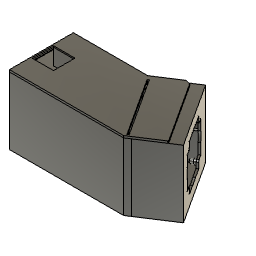
Spectroscope v11 (Autodesk Fusion 360 design; units mm, degrees)
Autodesk Fusion 360 part; units mm, degrees
(part 1 of 2)
sketch "Spectroscope Base" plane through (0, 0, 0) normal (0, 0, 1) x (1, 0, 0) in component "Spectrometer"
  line L0 (0, 0) -> (72, 0)
  line L1 (72, 0) -> (85.888295, -21.386099)
  line L2 (72, 0) -> (97.5, 0) construction
  line L3 (72, 0) -> (58.111705, 21.386099)
  line L4 (58.111705, 21.386099) -> (58.614907, 21.712883)
  line L5 (58.111705, 21.386099) -> (57.608502, 21.059316)
  line L6 (57.608502, 21.059316) -> (85.385093, -21.712883)
  line L7 (85.385093, -21.712883) -> (86.391498, -21.059316)
  line L8 (86.391498, -21.059316) -> (58.614907, 21.712883)
  line L9 (0, 0) -> (0, 23.787847)
  line L10 (0, 0) -> (0, -23.787847)
  line L11 (72, 0) -> (73.761208, 1.143742)
  line L12 (73.761208, 1.143742) -> (59.055954, 23.787847)
  line L13 (59.055954, 23.787847) -> (55.533538, 21.500363)
  line L14 (55.533538, 21.500363) -> (84.944046, -23.787847)
  line L15 (84.944046, -23.787847) -> (88.466462, -21.500363)
  line L16 (88.466462, -21.500363) -> (73.761208, 1.143742)
  line L17 (0, 23.787847) -> (59.055954, 23.787847)
  line L18 (0, -23.787847) -> (84.944046, -23.787847)
  line L19 (0, 0) -> (1.5, 0)
  line L20 (1.5, 0) -> (1.5, 22.287847)
  line L21 (1.5, 22.287847) -> (56.746157, 22.287847)
  line L22 (1.5, 0) -> (1.5, -22.287847)
  line L23 (1.5, -22.287847) -> (83.969934, -22.287847)
  line L24 (1.5, 0) -> (16.5, 0)
  line L25 (16.5, 0) -> (16.5, 7.5)
  line L26 (16.5, 7.5) -> (1.5, 7.5)
  line L27 (16.5, 0) -> (16.5, -7.5)
  line L28 (16.5, -7.5) -> (1.5, -7.5)
  line L29 (16.5, 0) -> (17.75, 0)
  line L30 (17.75, 0) -> (17.75, 8.75)
  line L31 (17.75, 8.75) -> (1.5, 8.75)
  line L32 (17.75, 0) -> (17.75, -8.75)
  line L33 (17.75, -8.75) -> (1.5, -8.75)
  line L34 (1.5, 0) -> (1.5, 1.469227)
  line L35 (1.5, 0) -> (1.5, 0.5)
  line L36 (1.5, 0.5) -> (0, 0.5)
  line L37 (1.5, 0) -> (1.5, -0.5)
  line L38 (1.5, -0.5) -> (0, -0.5)
  line L39 (0, -0.5) -> (0, 0.5)
  line L40 (58.111705, 21.386099) -> (60.8349, 17.192747)
  line L41 (60.8349, 17.192747) -> (62.596108, 18.336489)
  line L42 (60.8349, 17.192747) -> (59.073692, 16.049005)
  line L43 (85.888295, -21.386099) -> (83.1651, -17.192747)
  line L44 (83.1651, -17.192747) -> (81.403892, -18.336489)
  line L45 (83.1651, -17.192747) -> (84.926308, -16.049005)
  line L46 (55.533538, 21.500363) -> (55.02214, 22.287847)
  dimension "d1" = 72
  dimension "d3" = 25.5
  dimension "d4" = 25.5
  dimension "d9" = 123
  dimension "d10" = 0.6
  dimension "d11" = 0.6
  dimension "d12" = 51
  dimension "d13" = 1.2
  dimension "d14" = 51
  dimension "d18" = 23.787847
  dimension "d19" = 23.787847
  dimension "d22" = 2.1
  dimension "d23" = 27
  dimension "d24" = 4.2
  dimension "d25" = 90
  dimension "d26" = 54
  dimension "d27" = 4.2
  dimension "d28" = 27
  dimension "d29" = 1.5
  dimension "d30" = 22.287847
  dimension "d31" = 90
  dimension "d32" = 22.287847
  dimension "d34" = 15
  dimension "d35" = 7.5
  dimension "d36" = 15
  dimension "d37" = 7.5
  dimension "d38" = 15
  dimension "d40" = 1.25
  dimension "d41" = 8.75
  dimension "d42" = 16.25
  dimension "d43" = 8.75
  dimension "d44" = 16.25
  dimension "d46" = 0.5
  dimension "d47" = 1.5
  dimension "d48" = 0.5
  dimension "d49" = 1.5
  dimension "d50" = 1
  dimension "d52" = 5
  dimension "d53" = 2.1
  dimension "d54" = 2.1
  dimension "d55" = 5
  dimension "d56" = 2.1
  dimension "d57" = 2.1
  constraint coincident L0.start L9.start
  constraint horizontal L0
  constraint horizontal L2
  constraint parallel L1 L3
  constraint perpendicular L3 L4
  constraint perpendicular L3 L5
  constraint perpendicular L5 L6
  constraint perpendicular L1 L7
  constraint perpendicular L4 L8
  constraint perpendicular L0 L9
  constraint perpendicular L0 L10
  constraint perpendicular L6 L11
  constraint perpendicular L11 L12
  constraint perpendicular L13 L14
  constraint perpendicular L14 L15
  constraint perpendicular L11 L16
  constraint perpendicular L9 L19
  constraint perpendicular L17 L20
  constraint perpendicular L0 L22
  constraint horizontal L23
  constraint horizontal L24
  constraint vertical L25
  constraint horizontal L26
  constraint perpendicular L24 L27
  constraint perpendicular L27 L28
  constraint perpendicular L25 L29
  constraint perpendicular L29 L30
  constraint perpendicular L20 L31
  constraint perpendicular L29 L32
  constraint perpendicular L22 L33
  constraint perpendicular L19 L35
  constraint perpendicular L9 L36
  constraint perpendicular L36 L37
  constraint perpendicular L10 L38
  constraint perpendicular L36 L39
  constraint perpendicular L5 L40
  constraint perpendicular L12 L41
  constraint perpendicular L6 L42
  constraint perpendicular L7 L43
  constraint perpendicular L6 L44
  constraint perpendicular L43 L45
  constraint perpendicular L13 L46
  measures "d1" distance of L0.start L0.end
  measures "d9" angle of L0 L1
  measures "d25" angle of L12 L13
  measures "d29" distance of L0.start L19.end
  measures "d31" angle of L20 L21
  measures "d34" distance of L19.end L24.end
  measures "d35" distance of L24.end L25.end
  measures "d36" distance of L25.end L26.end
  measures "d37" distance of L24.end L27.end
  measures "d38" distance of L27.end L28.end
  measures "d40" distance of L24.end L29.end
  measures "d41" distance of L29.end L30.end
  measures "d42" distance of L30.end L31.end
  measures "d43" distance of L29.end L32.end
  measures "d44" distance of L32.end L33.end
  measures "d46" distance of L19.end L35.end
  measures "d47" distance of L35.end L36.end
  measures "d48" distance of L19.end L37.end
  measures "d49" distance of L37.end L38.end
  measures "d50" distance of L38.end L36.end
sketch "Sketch2" plane through (0, 0, 0) normal (1, 0, 0) x (0, 1, 0) in component "Spectrometer"
  line L0 (0, 0) -> (0, 50)
  line L1 (0, 50) -> (23.787847, 50)
  line L2 (0, 50) -> (-23.787847, 50)
  line L3 (-23.787847, 50) -> (-23.787847, 0)
  line L4 (23.787847, 50) -> (23.787847, 0)
  line L5 (23.787847, 0) -> (-23.787847, 0)
  line L6 (0, 0) -> (0, 1.5)
  dimension "d62" = 50
  dimension "d63" = 23.787847
  dimension "d64" = 23.787847
  dimension "d65" = 50
  dimension "d66" = 50
  dimension "d67" = 47.575695
  dimension "d68" = 1.5
  constraint coincident L0.start L6.start
  constraint vertical L0
  constraint perpendicular L0 L1
  constraint perpendicular L0 L2
  constraint perpendicular L2 L3
  constraint perpendicular L1 L4
  constraint perpendicular L4 L5
  constraint perpendicular L5 L6
  measures "d62" distance of L0.start L0.end
  measures "d68" distance of L0.start L6.end
ref_plane "WorkPlane1" through (71.496798, -0.326783, 0) normal (-0.838671, -0.544639, 0) x (0.544639, -0.838671, 0) in component "Spectrometer"
sketch "Camera Mount" plane through (71.496798, -0.326783, 0) normal (-0.838671, -0.544639, 0) x (0.544639, -0.838671, 0) in component "Spectrometer"
  line L0 (0, 0) -> (-27, 0)
  line L1 (0, 0) -> (0, 25)
  line L2 (0, 25) -> (14.000714, 39.000714)
  line L3 (0, 25) -> (19.8, 25) construction
  circle A0 centre (14.000714, 39.000714) radius 1.25
  line L4 (14.000714, 39.000714) -> (16.998847, 41.998847)
  circle A1 centre (16.998847, 41.998847) radius 1.25
  circle A2 centre (-16.998847, 41.998847) radius 1.25
  line L5 (-14.000714, 39.000714) -> (-16.998847, 41.998847)
  circle A3 centre (-14.000714, 39.000714) radius 1.25
  line L6 (0, 25) -> (-14.000714, 39.000714)
  circle A4 centre (-16.998847, 8.001153) radius 1.25
  line L7 (-14.000714, 10.999286) -> (-16.998847, 8.001153)
  circle A5 centre (-14.000714, 10.999286) radius 1.25
  line L8 (0, 25) -> (-14.000714, 10.999286)
  circle A6 centre (16.998847, 8.001153) radius 1.25
  line L9 (14.000714, 10.999286) -> (16.998847, 8.001153)
  circle A7 centre (14.000714, 10.999286) radius 1.25
  line L10 (0, 25) -> (14.000714, 10.999286)
  line L11 (-19.5, 5.5) -> (19.5, 5.5)
  line L12 (19.5, 5.5) -> (19.5, 44.5)
  line L13 (19.5, 44.5) -> (-19.5, 44.5)
  line L14 (-19.5, 44.5) -> (-19.5, 5.5)
  line L15 (-19.5, 5.5) -> (19.5, 44.5) construction
  line L16 (19.5, 5.5) -> (-19.5, 44.5) construction
  line L17 (27, 50) -> (-27, 50)
  line L18 (-27, 50) -> (-27, 0)
  line L19 (-27, 0) -> (27, 0)
  line L20 (27, 0) -> (27, 50)
  line L21 (27, 50) -> (-27, 0) construction
  line L22 (-27, 50) -> (27, 0) construction
  circle A8 centre (16.998847, 41.998847) radius 1.75
  circle A9 centre (14.000714, 39.000714) radius 1.75
  circle A10 centre (-16.998847, 41.998847) radius 1.75
  circle A11 centre (-14.000714, 39.000714) radius 1.75
  circle A12 centre (-16.998847, 8.001153) radius 1.75
  circle A13 centre (-14.000714, 10.999286) radius 1.75
  circle A14 centre (16.998847, 8.001153) radius 1.75
  circle A15 centre (14.000714, 10.999286) radius 1.75
  line L23 (-14.000714, 10.999286) -> (-6.750714, 10.999286)
  line L24 (-11.750714, 7.999286) -> (-1.750714, 7.999286)
  line L25 (-1.750714, 7.999286) -> (-1.750714, 13.999286)
  line L26 (-1.750714, 13.999286) -> (-11.750714, 13.999286)
  line L27 (-11.750714, 13.999286) -> (-11.750714, 7.999286)
  line L28 (-11.750714, 7.999286) -> (-1.750714, 13.999286) construction
  line L29 (-1.750714, 7.999286) -> (-11.750714, 13.999286) construction
  line L30 (-17.000714, 13.249286) -> (-11.000714, 23.249286) construction
  line L31 (-11.000714, 13.249286) -> (-17.000714, 13.249286)
  line L32 (-11.000714, 23.249286) -> (-11.000714, 13.249286)
  line L33 (-17.000714, 23.249286) -> (-11.000714, 13.249286) construction
  line L34 (-17.000714, 13.249286) -> (-17.000714, 23.249286)
  line L35 (-17.000714, 23.249286) -> (-11.000714, 23.249286)
  line L36 (-14.000714, 10.999286) -> (-14.000714, 18.249286)
  line L37 (-11.750714, 13.999286) -> (-11.000714, 14.749286)
  line L38 (-11.750714, 13.999286) -> (-10.690054, 13.999286) construction
  line L39 (-11.750714, 13.999286) -> (-12.500714, 13.249286)
  line L40 (-11.000714, 13.249286) -> (-10.250714, 13.999286)
  line L41 (-11.000714, 13.249286) -> (-11.750714, 12.499286)
  line L42 (11.750714, 7.999286) -> (1.750714, 13.999286) construction
  line L43 (11.000714, 23.249286) -> (11.000714, 13.249286)
  line L44 (17.000714, 23.249286) -> (11.000714, 13.249286) construction
  line L45 (11.000714, 13.249286) -> (11.000714, 14.309946) construction
  line L46 (11.750714, 7.999286) -> (1.750714, 7.999286)
  line L47 (11.000714, 13.249286) -> (17.000714, 13.249286)
  line L48 (-25, 52) -> (25, -2) construction
  line L49 (11.000714, 13.249286) -> (10.250714, 13.999286)
  line L50 (14.000714, 10.999286) -> (6.750714, 10.999286)
  line L51 (0, 25) -> (14.000714, 10.999286)
  line L52 (19.5, 5.5) -> (-19.5, 44.5) construction
  line L53 (1.750714, 7.999286) -> (1.750714, 13.999286)
  line L54 (1.750714, 13.999286) -> (11.750714, 13.999286)
  line L55 (11.000714, 13.249286) -> (11.750714, 12.499286)
  line L56 (11.750714, 13.999286) -> (11.750714, 7.999286)
  line L57 (1.750714, 7.999286) -> (11.750714, 13.999286) construction
  line L58 (11.750714, 13.999286) -> (11.000714, 14.749286)
  line L59 (17.000714, 13.249286) -> (17.000714, 23.249286)
  line L60 (14.000714, 10.999286) -> (14.000714, 18.249286)
  line L61 (17.000714, 13.249286) -> (11.000714, 23.249286) construction
  line L62 (17.000714, 23.249286) -> (11.000714, 23.249286)
  line L63 (11.750714, 13.999286) -> (12.500714, 13.249286)
  line L64 (17.000714, 36.750714) -> (11.000714, 26.750714) construction
  line L65 (1.750714, 36.000714) -> (11.750714, 36.000714)
  line L66 (1.750714, 42.000714) -> (11.750714, 36.000714) construction
  line L67 (11.750714, 36.000714) -> (10.690054, 36.000714) construction
  line L68 (17.000714, 36.750714) -> (17.000714, 26.750714)
  line L69 (11.750714, 36.000714) -> (11.750714, 42.000714)
  line L70 (-27, 0) -> (27, 50) construction
  line L71 (11.750714, 36.000714) -> (11.000714, 35.250714)
  line L72 (14.000714, 39.000714) -> (14.000714, 31.750714)
  line L73 (0, 25) -> (14.000714, 39.000714)
  line L74 (19.5, 44.5) -> (-19.5, 5.5) construction
  line L75 (17.000714, 26.750714) -> (11.000714, 26.750714)
  line L76 (11.000714, 26.750714) -> (11.000714, 36.750714)
  line L77 (11.750714, 36.000714) -> (12.500714, 36.750714)
  line L78 (11.000714, 36.750714) -> (17.000714, 36.750714)
  line L79 (17.000714, 26.750714) -> (11.000714, 36.750714) construction
  line L80 (11.000714, 36.750714) -> (10.250714, 36.000714)
  line L81 (11.750714, 42.000714) -> (1.750714, 42.000714)
  line L82 (14.000714, 39.000714) -> (6.750714, 39.000714)
  line L83 (11.750714, 42.000714) -> (1.750714, 36.000714) construction
  line L84 (1.750714, 42.000714) -> (1.750714, 36.000714)
  line L85 (11.000714, 36.750714) -> (11.750714, 37.500714)
  line L86 (-11.750714, 42.000714) -> (-1.750714, 36.000714) construction
  line L87 (-11.000714, 26.750714) -> (-11.000714, 36.750714)
  line L88 (-17.000714, 26.750714) -> (-11.000714, 36.750714) construction
  line L89 (-11.000714, 36.750714) -> (-11.000714, 35.690054) construction
  line L90 (-11.750714, 42.000714) -> (-1.750714, 42.000714)
  line L91 (-11.000714, 36.750714) -> (-17.000714, 36.750714)
  line L92 (25, -2) -> (-25, 52) construction
  line L93 (-11.000714, 36.750714) -> (-10.250714, 36.000714)
  line L94 (-14.000714, 39.000714) -> (-6.750714, 39.000714)
  line L95 (0, 25) -> (-14.000714, 39.000714)
  line L96 (-19.5, 44.5) -> (19.5, 5.5) construction
  line L97 (-1.750714, 42.000714) -> (-1.750714, 36.000714)
  line L98 (-1.750714, 36.000714) -> (-11.750714, 36.000714)
  line L99 (-11.000714, 36.750714) -> (-11.750714, 37.500714)
  line L100 (-11.750714, 36.000714) -> (-11.750714, 42.000714)
  line L101 (-1.750714, 42.000714) -> (-11.750714, 36.000714) construction
  line L102 (-11.750714, 36.000714) -> (-11.000714, 35.250714)
  line L103 (-17.000714, 36.750714) -> (-17.000714, 26.750714)
  line L104 (-14.000714, 39.000714) -> (-14.000714, 31.750714)
  line L105 (-17.000714, 36.750714) -> (-11.000714, 26.750714) construction
  line L106 (-17.000714, 26.750714) -> (-11.000714, 26.750714)
  line L107 (-11.750714, 36.000714) -> (-12.500714, 36.750714)
  point P0 (0, 25)
  point P1 (0, 25)
  point P2 (-6.750714, 10.999286)
  point P3 (-14.000714, 18.249286)
  point P4 (6.750714, 10.999286)
  point P5 (14.000714, 18.249286)
  point P6 (14.000714, 31.750714)
  point P7 (6.750714, 39.000714)
  point P8 (-6.750714, 39.000714)
  point P9 (-14.000714, 31.750714)
  dimension "d70" = 27
  dimension "d71" = 25
  dimension "d73" = 45
  dimension "d74" = 19.8
  dimension "d80" = 2.5
  dimension "d82" = 4.24
  dimension "d83" = 2.5
  dimension "d85" = 360
  dimension "d87" = 39
  dimension "d88" = 39
  dimension "d89" = 54
  dimension "d90" = 50
  dimension "d92" = 3.5
  dimension "d93" = 3.5
  dimension "d95" = 360
  dimension "d96" = 7.25
  dimension "d97" = 10
  dimension "d98" = 6
  dimension "d99" = 45
  dimension "d101" = 360
  constraint coincident L0.start L1.start
  constraint horizontal L0
  constraint perpendicular L0 L1
  constraint horizontal L3
  constraint parallel L2 L4
  constraint horizontal L11
  constraint perpendicular L11 L12
  constraint parallel L11 L13
  constraint parallel L12 L14
  constraint coincident L15 P1
  constraint coincident L16 P1
  constraint coincident P1 P0
  constraint horizontal L17
  constraint perpendicular L17 L18
  constraint parallel L17 L19
  constraint parallel L18 L20
  constraint coincident L21 P1
  constraint coincident L22 P1
  constraint horizontal L23
  constraint horizontal L24
  constraint perpendicular L24 L25
  constraint parallel L24 L26
  constraint parallel L25 L27
  constraint horizontal L38
  constraint parallel L37 L39
  constraint parallel L39 L40
  constraint parallel L40 L41
  measures "d70" distance of L0.start L0.end
  measures "d71" distance of L0.start P0
  measures "d73" angle of L2 L3
  measures "d80" diameter of A0
  measures "d83" diameter of A1
  measures "d87" distance of L12.end L13.end
  measures "d88" distance of L11.end L12.end
  measures "d89" distance of L0.end L19.end
  measures "d90" distance of L17.end L0.end
  measures "d92" diameter of A8
  measures "d93" diameter of A9
  measures "d99" angle of L37 L38
extrude "Extrude1" add sketch "Spectroscope Base" along normal blind 1.5 contours L0 L9 L19 L20 L34 L35 L36 L39 | L0 L10 L19 L22 L37 L38 L39 | L0 L20 L24 L25 L26 L34 L35 | L0 L22 L24 L27 L28 L37 | L9 L13 L17 L20 L21 L34 L36 | L10 L14 L18 L22 L23 L38 | L0 L20 L25 L26 L29 L30 L31 | L0 L22 L27 L28 L29 L32 L33 | L0 L14 L20 L21 L30 L31 L46 | L0 L14 L22 L23 L32 L33 | L4 L5 L6 L8 L12 L13 L14 L41 L42 | L6 L7 L8 L14 L15 L16 L44 L45 | L0 L6 L14 L42 | L0 L6 L14 L44 | L8 L11 L12 L41 | L13 L21 L46 | L0 L3 L6 L42 | L0 L1 L6 L44 | L8 L11 L16 L45 | L3 L4 L8 L40 L41 | L3 L8 L11 L41 | L1 L8 L11 L45 | L3 L5 L6 L40 L42 | L1 L6 L7 L43 L44 | L1 L7 L8 L43 L45 picked at (0.5, 0.333333) picked at (0.5, -0.333333) picked at (11.5, 2.989742) picked at (11.5, -2.666667) picked at (0.5, 11.012616) picked at (28.814682, -23.287847) picked at (11.916667, 8.333333) picked at (11.916667, -8.333333) picked at (48.773243, 5.349668) picked at (56.216643, -9.02883) picked at (60.08899, 21.279073) picked at (86.594756, -19.536228) picked at (67.037439, 5.621988) picked at (74.061504, -6.112163) picked at (69.200838, 6.330018) picked at (55.767278, 22.025353) picked at (68.039827, 5.730916) picked at (75.315493, -5.839843) picked at (80.785273, -10.590409) picked at (60.094902, 18.699459) picked at (64.892068, 11.679687) picked at (75.889434, -5.621988) picked at (58.851702, 19.879387) picked at (83.905098, -18.699459) picked at (85.316032, -19.77046) makes body 1 in component "Spectrometer"
extrude "Extrude2" add sketch "Spectroscope Base" along normal blind 50 separate body contours L0 L9 L19 L20 L34 L35 L36 L39 | L0 L10 L19 L22 L37 L38 L39 | L9 L13 L17 L20 L21 L34 L36 | L10 L14 L18 L22 L23 L38 | L4 L5 L6 L8 L12 L13 L14 L41 L42 | L6 L7 L8 L14 L15 L16 L44 L45 | L13 L21 L46 picked at (0.5, 0.333333) picked at (0.5, -0.333333) picked at (0.5, 11.012616) picked at (28.814682, -23.287847) picked at (60.08899, 21.279073) picked at (86.594756, -19.536228) picked at (55.767278, 22.025353) makes body 2 in component "Spectrometer"
extrude "Extrude3" add sketch "Spectroscope Base" along normal blind 7.5 contours L0 L20 L25 L26 L29 L30 L31 | L0 L22 L27 L28 L29 L32 L33 | L0 L6 L14 L42 | L0 L6 L14 L44 | L8 L11 L12 L41 | L8 L11 L16 L45 picked at (11.916667, 8.333333) picked at (11.916667, -8.333333) picked at (67.037439, 5.621988) picked at (74.061504, -6.112163) picked at (69.200838, 6.330018) picked at (80.785273, -10.590409) bodies 1 2 in component "Spectrometer"
extrude "Extrude4" cut sketch "Spectroscope Base" along normal blind 12 from surface at 19 contours L0 L9 L19 L20 L34 L35 L36 L39 | L0 L10 L19 L22 L37 L38 L39 picked at (0.5, 0.333333) picked at (0.5, -0.333333) bodies 1 in component "Spectrometer"
extrude "Extrude5" add sketch "Camera Mount" along normal blind 1.5 separate body contours L0 L17 L18 L19 L20 | L2 L73 L76 L78 | L2 L65 L69 L73 | L65 L71 L76 | L65 L76 L80 | L2 A9 L69 L73 L82 | L69 L77 L78 | L69 L78 L85 | L2 A9 L72 L73 L78 | L2 A0 A9 L73 L82 | L2 A0 A9 L72 L73 | L2 A0 L73 L82 | L2 A0 L72 L73 | A0 L4 A9 L82 | A0 L4 A9 L72 | A0 L4 L82 | A0 L4 L72 | A1 | A2 | L5 A3 L104 | A3 L6 L94 L95 | L5 A3 L94 | A3 L6 L95 L104 | L5 A3 A11 L104 | L5 A3 A11 L94 | A3 L6 A11 L95 L104 | A3 L6 A11 L94 L95 | L6 A11 L94 L95 L100 | L6 A11 L91 L95 L104 | L6 L87 L91 L95 | L91 L99 L100 | L91 L100 L107 | L6 L95 L98 L100 | L87 L93 L98 | L87 L98 L102 | A4 | L7 A5 L23 | A5 L8 L36 | A5 L8 L23 | L7 A5 L36 | L7 A5 A13 L23 | L7 A5 A13 L36 | A5 L8 A13 L23 | A5 L8 A13 L36 | L8 A13 L31 L36 | L8 A13 L23 L27 | L8 L26 L27 | L27 L31 L39 | L27 L31 L41 | L8 L31 L32 | L26 L32 L37 | L26 L32 L40 | A6 | L9 A7 L60 | A7 L10 L50 L51 | L9 A7 L50 | A7 L10 L51 L60 | L9 A7 A15 L60 | L9 A7 A15 L50 | A7 L10 A15 L51 L60 | A7 L10 A15 L50 L51 | L10 A15 L50 L51 L56 | L10 A15 L47 L51 L60 | L10 L43 L47 L51 | L47 L55 L56 | L47 L56 L63 | L10 L51 L54 L56 | L43 L49 L54 | L43 L54 L58 | L11 L12 L13 L14 | A8 | A10 | A12 | A14 picked at (-24.5, 31.5) picked at (11.250714, 36.500714) picked at (11.500714, 36.250714) picked at (11.250714, 35.750714) picked at (10.750714, 36.250714) picked at (11.937258, 38.349736) picked at (12.000714, 36.500714) picked at (11.500714, 37.000714) picked at (13.349736, 36.937258) picked at (12.422371, 38.924574) picked at (13.924574, 37.422371) picked at (13.170946, 38.946328) picked at (13.946328, 38.170946) picked at (14.163585, 40.571634) picked at (15.47005, 38.420955) picked at (13.225327, 39.299814) picked at (14.812929, 38.824028) picked at (17.295564, 42.324189) picked at (-17.550973, 42.311234) picked at (-14.82554, 39.102447) picked at (-13.254921, 38.63293) picked at (-13.345539, 39.512018) picked at (-13.63293, 38.254921) picked at (-15.456712, 39.612586) picked at (-12.516447, 39.540406) picked at (-13.100286, 37.702179) picked at (-12.513378, 38.467053) picked at (-11.937258, 38.349736) picked at (-13.349736, 36.937258) picked at (-11.250714, 36.500714) picked at (-11.500714, 37.000714) picked at (-12.000714, 36.500714) picked at (-11.500714, 36.250714) picked at (-10.750714, 36.250714) picked at (-11.250714, 35.750714) picked at (-16.820738, 8.324208) picked at (-13.225327, 10.700186) picked at (-13.946328, 11.829054) picked at (-13.185143, 11.161513) picked at (-14.82554, 10.897553) picked at (-12.428204, 10.852555) picked at (-15.530734, 10.607676) picked at (-12.445813, 11.28079) picked at (-12.979474, 12.205118) picked at (-13.349736, 13.062742) picked at (-11.937258, 11.650264) picked at (-11.500714, 13.749286) picked at (-12.000714, 13.499286) picked at (-11.500714, 12.999286) picked at (-11.250714, 13.499286) picked at (-11.250714, 14.249286) picked at (-10.750714, 13.749286) picked at (17.345998, 8.256868) picked at (14.666132, 11.497411) picked at (13.213295, 11.266578) picked at (13.171891, 10.938148) picked at (13.63293, 11.745079) picked at (15.47005, 11.579045) picked at (12.428204, 10.852555) picked at (13.870188, 12.574064) picked at (12.445813, 11.28079) picked at (11.937258, 11.650264) picked at (13.349736, 13.062742) picked at (11.250714, 13.499286) picked at (11.500714, 12.999286) picked at (12.000714, 13.499286) picked at (11.500714, 13.749286) picked at (10.750714, 13.749286) picked at (11.250714, 14.249286) picked at (-0.583571, 20.165952) picked at (18.571357, 41.852117) picked at (-18.539622, 41.652291) picked at (-15.426533, 7.85311) picked at (17.299004, 9.551709) makes body 3 in component "Spectrometer"
extrude "Extrude6" add sketch "Camera Mount" along normal blind 3 contours L2 A0 A9 L73 L82 | L2 A0 A9 L72 L73 | L2 A0 L73 L82 | L2 A0 L72 L73 | A0 L4 A9 L82 | A0 L4 A9 L72 | A0 L4 L82 | A0 L4 L72 | A1 | A2 | L5 A3 L104 | A3 L6 L94 L95 | L5 A3 L94 | A3 L6 L95 L104 | L5 A3 A11 L104 | L5 A3 A11 L94 | A3 L6 A11 L95 L104 | A3 L6 A11 L94 L95 | A4 | L7 A5 L23 | A5 L8 L36 | A5 L8 L23 | L7 A5 L36 | L7 A5 A13 L23 | L7 A5 A13 L36 | A5 L8 A13 L23 | A5 L8 A13 L36 | A6 | L9 A7 L60 | A7 L10 L50 L51 | L9 A7 L50 | A7 L10 L51 L60 | L9 A7 A15 L60 | L9 A7 A15 L50 | A7 L10 A15 L51 L60 | A7 L10 A15 L50 L51 | A8 | A10 | A12 | A14 picked at (12.422371, 38.924574) picked at (13.924574, 37.422371) picked at (13.170946, 38.946328) picked at (13.946328, 38.170946) picked at (14.163585, 40.571634) picked at (15.47005, 38.420955) picked at (13.225327, 39.299814) picked at (14.812929, 38.824028) picked at (17.295564, 42.324189) picked at (-17.550973, 42.311234) picked at (-14.82554, 39.102447) picked at (-13.254921, 38.63293) picked at (-13.345539, 39.512018) picked at (-13.63293, 38.254921) picked at (-15.456712, 39.612586) picked at (-12.516447, 39.540406) picked at (-13.100286, 37.702179) picked at (-12.513378, 38.467053) picked at (-16.820738, 8.324208) picked at (-13.225327, 10.700186) picked at (-13.946328, 11.829054) picked at (-13.185143, 11.161513) picked at (-14.82554, 10.897553) picked at (-12.428204, 10.852555) picked at (-15.530734, 10.607676) picked at (-12.445813, 11.28079) picked at (-12.979474, 12.205118) picked at (17.345998, 8.256868) picked at (14.666132, 11.497411) picked at (13.213295, 11.266578) picked at (13.171891, 10.938148) picked at (13.63293, 11.745079) picked at (15.47005, 11.579045) picked at (12.428204, 10.852555) picked at (13.870188, 12.574064) picked at (12.445813, 11.28079) picked at (18.571357, 41.852117) picked at (-18.539622, 41.652291) picked at (-15.426533, 7.85311) picked at (17.299004, 9.551709) bodies 3 in component "Spectrometer"
extrude "Extrude7" add sketch "Camera Mount" along normal blind 5.5 contours L2 A0 L73 L82 | L2 A0 L72 L73 | A0 L4 L82 | A0 L4 L72 | A1 | A2 | L5 A3 L104 | A3 L6 L94 L95 | L5 A3 L94 | A3 L6 L95 L104 | A4 | L7 A5 L23 | A5 L8 L36 | A5 L8 L23 | L7 A5 L36 | A6 | L9 A7 L60 | A7 L10 L50 L51 | L9 A7 L50 | A7 L10 L51 L60 picked at (13.170946, 38.946328) picked at (13.946328, 38.170946) picked at (13.225327, 39.299814) picked at (14.812929, 38.824028) picked at (17.295564, 42.324189) picked at (-17.550973, 42.311234) picked at (-14.82554, 39.102447) picked at (-13.254921, 38.63293) picked at (-13.345539, 39.512018) picked at (-13.63293, 38.254921) picked at (-16.820738, 8.324208) picked at (-13.225327, 10.700186) picked at (-13.946328, 11.829054) picked at (-13.185143, 11.161513) picked at (-14.82554, 10.897553) picked at (17.345998, 8.256868) picked at (14.666132, 11.497411) picked at (13.213295, 11.266578) picked at (13.171891, 10.938148) picked at (13.63293, 11.745079) bodies 3 in component "Spectrometer"
chamfer "Chamfer1" distance 0.2 angle 45 8 edges at (58.624047, 9.397083, 10.547266) (56.991147, 11.911529, 7.549134) (73.874718, -14.086891, 10.547266) (75.507618, -16.601336, 7.549134) (73.874718, -14.086891, 38.548695) (75.507618, -16.601336, 41.546828) (56.991147, 11.911529, 41.546828) (58.624047, 9.397083, 38.548695) on bodies 3 in component "Spectrometer"
sketch "Camera Wall" plane through (71.496798, -0.326783, 0) normal (-0.838671, -0.544639, 0) x (0.544639, -0.838671, 0) in component "Spectrometer"
  line L0 (0, 0) -> (0, 25)
  line L1 (-27, 0) -> (27, 0)
  line L2 (27, 0) -> (27, 50)
  line L3 (27, 50) -> (-27, 50)
  line L4 (-27, 50) -> (-27, 0)
  line L5 (-27, 0) -> (27, 50) construction
  line L6 (27, 0) -> (-27, 50) construction
  line L7 (-25.5, 1.5) -> (25.5, 1.5)
  line L8 (25.5, 1.5) -> (25.5, 48.5)
  line L9 (25.5, 48.5) -> (-25.5, 48.5)
  line L10 (-25.5, 48.5) -> (-25.5, 1.5)
  line L11 (-25.5, 1.5) -> (25.5, 48.5) construction
  line L12 (25.5, 1.5) -> (-25.5, 48.5) construction
  line L13 (-25.5, 48.5) -> (-25.5, 50)
  line L14 (-25.5, 1.5) -> (-25.5, 0)
  line L15 (25.5, 1.5) -> (25.5, 0)
  line L16 (25.5, 48.5) -> (25.5, 50)
  line L17 (0, 25) -> (12.303658, 37.303658)
  line L18 (0, 25) -> (17.5, 25) construction
  circle A0 centre (0, 25) radius 17.4
  line L19 (25.5, 25) -> (24, 25)
  line L20 (24, 25) -> (25.5, 27.598076)
  line L21 (24, 25) -> (27, 25) construction
  line L22 (24, 25) -> (25.5, 22.401924)
  line L23 (-25.5, 25) -> (-24, 25)
  line L24 (-24, 25) -> (-25.5, 27.598076)
  line L25 (-24, 25) -> (-21, 25) construction
  line L26 (-24, 25) -> (-25.5, 22.401924)
  point P0 (0, 25)
  point P1 (0, 25)
  dimension "d120" = 25
  dimension "d121" = 54
  dimension "d122" = 50
  dimension "d123" = 51
  dimension "d124" = 47
  dimension "d155" = 45
  dimension "d156" = 17.4
  dimension "d157" = 34.8
  dimension "d201" = 1.5
  dimension "d202" = 60
  dimension "d203" = 60
  dimension "d204" = 1.5
  dimension "d205" = 120
  dimension "d206" = 60
  constraint coincident L0.start origin
  constraint vertical L0
  constraint horizontal L1
  constraint perpendicular L1 L2
  constraint parallel L1 L3
  constraint parallel L2 L4
  constraint coincident L5 P1
  constraint coincident L6 P1
  constraint coincident P1 P0
  constraint horizontal L7
  constraint perpendicular L7 L8
  constraint parallel L7 L9
  constraint parallel L8 L10
  constraint coincident L11 P1
  constraint coincident L12 P1
  constraint coincident L3 L13.end
  constraint perpendicular L3 L13
  constraint coincident L1 L14.end
  constraint perpendicular L1 L14
  constraint coincident L1 L15.end
  constraint perpendicular L1 L15
  constraint coincident L3 L16.end
  constraint perpendicular L3 L16
  constraint horizontal L18
  constraint midpoint L8 L19.start
  constraint perpendicular L8 L19
  constraint horizontal L21
  constraint midpoint L10 L23.start
  constraint perpendicular L10 L23
  constraint horizontal L25
  measures "d120" distance of L0.start P0
  measures "d121" distance of L2.end L3.end
  measures "d122" distance of L1.end L2.end
  measures "d123" distance of L8.end L9.end
  measures "d124" distance of L7.end L8.end
  measures "d155" angle of L17 L18
  measures "d157" diameter of A0
  measures "d201" distance of L19.start L19.end
  measures "d202" angle of L20 L21
  measures "d203" angle of L20 L22
  measures "d204" distance of L23.start L23.end
  measures "d205" angle of L24 L25
  measures "d206" angle of L24 L26
extrude "Extrude8" add sketch "Camera Wall" along normal blind 18 contours L0 L1 L7 L14 | L0 L1 L7 L15 | L1 L3 L4 L10 L13 L14 | L1 L2 L3 L8 L15 L16 | L10 L23 L26 | L8 L19 L22 | L10 L23 L24 | L8 L19 L20 | L3 L9 L13 L16 picked at (-17, 0.5) picked at (17, 1) picked at (-26.5, 25.866025) picked at (26.5, 25) picked at (-25, 24.133975) picked at (25, 24.133975) picked at (-25, 25.866025) picked at (25, 25.866025) picked at (8.5, 49) bodies 3 in component "Spectrometer"
move_body "Move1" bodies 3 to x (1, 0, 0) y (0, 1, 0) z (0, 0, 1) at (25.747186, 16.720418, 0) in component "Spectrometer"
extrude "Extrude9" add sketch "Spectroscope Base" along normal blind 1.5 from surface at 50 separate body contours L0 L9 L19 L20 L34 L35 L36 L39 | L0 L10 L19 L22 L37 L38 L39 | L9 L13 L17 L20 L21 L34 L36 | L10 L14 L18 L22 L23 L38 | L0 L20 L25 L26 L29 L30 L31 | L0 L22 L27 L28 L29 L32 L33 | L0 L14 L20 L21 L30 L31 L46 | L0 L14 L22 L23 L32 L33 | L4 L5 L6 L8 L12 L13 L14 L41 L42 | L6 L7 L8 L14 L15 L16 L44 L45 | L0 L6 L14 L42 | L0 L6 L14 L44 | L8 L11 L12 L41 | L13 L21 L46 | L8 L11 L16 L45 picked at (0.5, 0.333333) picked at (0.5, -0.333333) picked at (0.5, 11.012616) picked at (28.814682, -23.287847) picked at (11.916667, 8.333333) picked at (11.916667, -8.333333) picked at (48.773243, 5.349668) picked at (56.216643, -9.02883) picked at (60.08899, 21.279073) picked at (86.594756, -19.536228) picked at (67.037439, 5.621988) picked at (74.061504, -6.112163) picked at (69.200838, 6.330018) picked at (55.767278, 22.025353) picked at (80.785273, -10.590409) makes body 4 in component "Spectrometer"
extrude "Extrude10" add sketch "Spectroscope Base" against normal blind 1.5 from surface at 50 contours L0 L20 L25 L26 L29 L30 L31 | L0 L22 L27 L28 L29 L32 L33 | L0 L14 L20 L21 L30 L31 L46 | L0 L14 L22 L23 L32 L33 picked at (11.916667, 8.333333) picked at (11.916667, -8.333333) picked at (48.773243, 5.349668) picked at (56.216643, -9.02883) bodies 4 in component "Spectrometer"
extrude "Extrude11" add sketch "Spectroscope Base" against normal blind 10 from surface at 48.5 contours L0 L20 L25 L26 L29 L30 L31 | L0 L22 L27 L28 L29 L32 L33 picked at (11.916667, 8.333333) picked at (11.916667, -8.333333) bodies 4 in component "Spectrometer"
chamfer "Chamfer2" distance 0.5 angle 45 5 edges at (1.5, 0, 50) (42.734967, -22.287847, 50) (28.26107, 22.287847, 50) (57.047916, 19.168426, 50) (82.686913, -20.312168, 50) on bodies 1 in component "Spectrometer"
chamfer "Chamfer2" distance 0.5 angle 45 3 edges at (9, -7.5, 7.5) (16.5, 0, 7.5) (9, 7.5, 7.5) on bodies 1 in component "Spectrometer"
chamfer "Chamfer3" distance 0.5 angle 45 11 edges at (28.26107, 22.287847, 48.5) (69.496037, 0, 48.5) (42.734967, -22.287847, 48.5) (1.5, 15.518924, 48.5) (1.5, -15.518924, 48.5) (1.5, 8.125, 38.5) (1.5, -8.125, 38.5) (9, -7.5, 51.5) (16.5, 0, 51.5) (9, 7.5, 51.5) (1.5, 0, 51.5) on bodies 4 in component "Spectrometer"
extrude "Extrude12" add 1 faces at (77.482908, -4.587174, 2.5) along direction (0.83867057, 0.54463904, 0) blind 10 on bodies 1 bodies 1 in component "Spectrometer"
extrude "Extrude13" cut sketch "Camera Wall" along normal blind 10 from surface at -12.7 contours L1 L3 L4 L10 L13 L14 | L1 L2 L3 L8 L15 L16 | L10 L23 L26 | L8 L19 L22 | L10 L23 L24 | L8 L19 L20 picked at (-26.5, 25.866025) picked at (26.5, 25) picked at (-25, 24.133975) picked at (25, 24.133975) picked at (-25, 25.866025) picked at (25, 25.866025) bodies 1 in component "Spectrometer"
extrude "Extrude14" add sketch "Camera Wall" along normal blind 10 from surface at -12.7 contours L1 L3 L4 L10 L13 L14 | L1 L2 L3 L8 L15 L16 | L10 L23 L26 | L8 L19 L22 | L10 L23 L24 | L8 L19 L20 picked at (-26.5, 25.866025) picked at (26.5, 25) picked at (-25, 24.133975) picked at (25, 24.133975) picked at (-25, 25.866025) picked at (25, 25.866025) bodies 3 in component "Spectrometer"
chamfer "Chamfer4" distance 0.5 angle 45 4 edges at (96.036209, -14.795967, 11.200962) (96.036209, -14.795967, 38.799038) (68.259618, 27.976232, 38.799038) (68.259618, 27.976232, 11.200962) on bodies 1 in component "Spectrometer"
chamfer "Chamfer4" distance 0.5 angle 45 4 edges at (68.668098, 27.347229, 26.299038) (68.668098, 27.347229, 23.700962) (95.62773, -14.166964, 26.299038) (95.62773, -14.166964, 23.700962) on bodies 1 in component "Spectrometer"
chamfer "Chamfer5" distance 0.5 angle 45 4 edges at (87.649504, -20.242358, 38.799038) (87.649504, -20.242358, 11.200962) (59.872913, 22.529841, 38.799038) (59.872913, 22.529841, 11.200962) on bodies 3 in component "Spectrometer"
chamfer "Chamfer5" distance 0.5 angle 45 4 edges at (60.281392, 21.900839, 26.299038) (60.281392, 21.900839, 23.700962) (87.241024, -19.613355, 23.700962) (87.241024, -19.613355, 26.299038) on bodies 3 in component "Spectrometer"
extrude "Extrude15" add 1 faces at (78.66296, -6.404293, 51) along direction (0.83867057, 0.54463904, 0) blind 20 on bodies 4 bodies 4 in component "Spectrometer"
chamfer "Chamfer6" distance 0.5 angle 45 2 edges at (105.239873, -10.607583, 50.75) (75.829366, 34.680628, 50.75) on bodies 4 in component "Spectrometer"
copy_body "CopyPasteBodies1" bodies 3 makes body 5 in component "Spectrometer"
extrude "Extrude16" cut sketch "Camera Wall" against normal blind 35.2 contours L0 L17 A0 | L0 L17 A0 picked at (-5.638338, 14.897586) picked at (11.540964, 24.174574) bodies 5 in component "Spectrometer"
chamfer "Chamfer7" distance 0.5 angle 45 3 edges at (9.25, 7.5, 38.5) (16.5, 0, 38.5) (9.25, -7.5, 38.5) on bodies 4 in component "Spectrometer"
copy_body "CopyPasteBodies2" bodies 1 makes body 6 in component "Spectrometer"
sketch "Modular Slit" plane through (0, 0, 0) normal (1, 0, 0) x (0, 1, 0) in component "Spectrometer"
  line L0 (0, 0) -> (-23.787847, 0)
  line L1 (-23.787847, 0) -> (-23.787847, 50)
  line L2 (-23.787847, 50) -> (23.787847, 50)
  line L3 (23.787847, 50) -> (23.787847, 0)
  line L4 (23.787847, 0) -> (0, 0)
  line L5 (0, 0) -> (0, 25)
  line L6 (-5, 17.5) -> (5, 17.5)
  line L7 (5, 17.5) -> (5, 32.5)
  line L8 (5, 32.5) -> (-5, 32.5)
  line L9 (-5, 32.5) -> (-5, 17.5)
  line L10 (-5, 17.5) -> (5, 32.5) construction
  line L11 (5, 17.5) -> (-5, 32.5) construction
  line L12 (0, 25) -> (-10, 25)
  line L13 (0, 25) -> (10, 25)
  line L14 (-7.5, 30) -> (-12.5, 30)
  line L15 (-12.5, 30) -> (-12.5, 20)
  line L16 (-12.5, 20) -> (-7.5, 20)
  line L17 (-7.5, 20) -> (-7.5, 30)
  line L18 (-7.5, 30) -> (-12.5, 20) construction
  line L19 (-12.5, 30) -> (-7.5, 20) construction
  line L20 (12.5, 20) -> (7.5, 20)
  line L21 (7.5, 20) -> (7.5, 30)
  line L22 (7.5, 30) -> (12.5, 30)
  line L23 (12.5, 30) -> (12.5, 20)
  line L24 (12.5, 20) -> (7.5, 30) construction
  line L25 (7.5, 20) -> (12.5, 30) construction
  line L26 (22.287847, 48.5) -> (-22.287847, 48.5)
  line L27 (-22.287847, 48.5) -> (-22.287847, 1.5)
  line L28 (-22.287847, 1.5) -> (22.287847, 1.5)
  line L29 (22.287847, 1.5) -> (22.287847, 48.5)
  line L30 (22.287847, 48.5) -> (-22.287847, 1.5) construction
  line L31 (-22.287847, 48.5) -> (22.287847, 1.5) construction
  line L32 (22.287847, 48.5) -> (17.287847, 48.5)
  line L33 (17.287847, 48.5) -> (17.287847, 47)
  line L34 (22.287847, 48.5) -> (22.287847, 43.5)
  line L35 (22.287847, 43.5) -> (20.787847, 43.5)
  line L36 (17.287847, 47) -> (20.787847, 47)
  line L37 (20.787847, 43.5) -> (20.787847, 47)
  line L38 (0, 25) -> (-2, 25)
  line L39 (0, 25) -> (0, 27)
  line L40 (-22.287847, 48.5) -> (-17.287847, 48.5)
  line L41 (-17.287847, 48.5) -> (-17.287847, 47)
  line L42 (-17.287847, 47) -> (-20.787847, 47)
  line L43 (-22.287847, 43.5) -> (-20.787847, 43.5)
  line L44 (-20.787847, 43.5) -> (-20.787847, 47)
  line L45 (-22.287847, 48.5) -> (-22.287847, 43.5)
  line L46 (22.287847, 1.5) -> (17.287847, 1.5)
  line L47 (22.287847, 6.5) -> (20.787847, 6.5)
  line L48 (20.787847, 6.5) -> (20.787847, 3)
  line L49 (17.287847, 1.5) -> (17.287847, 3)
  line L50 (22.287847, 1.5) -> (22.287847, 6.5)
  line L51 (17.287847, 3) -> (20.787847, 3)
  line L52 (-17.287847, 3) -> (-20.787847, 3)
  line L53 (-22.287847, 1.5) -> (-22.287847, 6.5)
  line L54 (-22.287847, 1.5) -> (-17.287847, 1.5)
  line L55 (-17.287847, 1.5) -> (-17.287847, 3)
  line L56 (-22.287847, 6.5) -> (-20.787847, 6.5)
  line L57 (-20.787847, 6.5) -> (-20.787847, 3)
  line L58 (-0.5, 19) -> (0.5, 19)
  line L59 (0.5, 19) -> (0.5, 31)
  line L60 (0.5, 31) -> (-0.5, 31)
  line L61 (-0.5, 31) -> (-0.5, 19)
  line L62 (-0.5, 19) -> (0.5, 31) construction
  line L63 (0.5, 19) -> (-0.5, 31) construction
  point P0 (0, 25)
  point P1 (-10, 25)
  point P2 (10, 25)
  point P3 (0, 25)
  point P4 (-22.287847, 1.5)
  point P5 (0, 25)
  dimension "d161" = 23.787847
  dimension "d162" = 50
  dimension "d163" = 47.575695
  dimension "d164" = 50
  dimension "d165" = 23.787847
  dimension "d166" = 25
  dimension "d167" = 10
  dimension "d168" = 15
  dimension "d169" = 10
  dimension "d170" = 10
  dimension "d174" = 5
  dimension "d175" = 10
  dimension "d176" = 5
  dimension "d177" = 10
  dimension "d178" = 44.575695
  dimension "d179" = 47
  dimension "d180" = 5
  dimension "d181" = 1.5
  dimension "d182" = 5
  dimension "d183" = 1.5
  dimension "d184" = 2
  dimension "d185" = 2
  dimension "d194" = 1
  dimension "d195" = 12
  constraint coincident L0.start L4.end
  constraint horizontal L0
  constraint perpendicular L0 L1
  constraint perpendicular L1 L2
  constraint perpendicular L2 L3
  constraint perpendicular L3 L4
  constraint perpendicular L0 L5
  constraint horizontal L6
  constraint perpendicular L6 L7
  constraint parallel L6 L8
  constraint parallel L7 L9
  constraint coincident L10 P5
  constraint coincident L11 P5
  constraint coincident P5 P3
  constraint perpendicular L9 L12
  constraint perpendicular L7 L13
  constraint horizontal L14
  constraint perpendicular L14 L15
  constraint parallel L14 L16
  constraint parallel L15 L17
  constraint coincident L18 P1
  constraint coincident L19 P1
  constraint coincident P1 L12.end
  constraint horizontal L20
  constraint perpendicular L20 L21
  constraint parallel L20 L22
  constraint parallel L21 L23
  constraint coincident L24 P2
  constraint coincident L25 P2
  constraint coincident P2 L13.end
  constraint horizontal L26
  constraint perpendicular L26 L27
  constraint parallel L26 L28
  constraint parallel L27 L29
  constraint coincident L30 P5
  constraint coincident L31 P5
  constraint perpendicular L29 L32
  constraint perpendicular L32 L33
  constraint perpendicular L26 L34
  constraint perpendicular L34 L35
  constraint vertical L37
  constraint perpendicular L36 L37
  constraint parallel L12 L38
  constraint perpendicular L38 L39
  constraint horizontal L58
  constraint perpendicular L58 L59
  constraint parallel L58 L60
  constraint parallel L59 L61
  constraint coincident L62 P5
  constraint coincident L63 P5
  measures "d166" distance of L0.start P5
  measures "d167" distance of L7.end L8.end
  measures "d168" distance of L6.end L7.end
  measures "d169" distance of P5 P1
  measures "d170" distance of P5 P2
  measures "d174" distance of L15.end L16.end
  measures "d175" distance of L14.end L15.end
  measures "d176" distance of L21.end L22.end
  measures "d177" distance of L20.end L21.end
  measures "d184" distance of P5 L38.end
  measures "d185" distance of P5 L39.end
  measures "d194" distance of L59.end L60.end
  measures "d195" distance of L58.end L59.end
extrude "Extrude17" cut sketch "Modular Slit" along normal blind 1.5 contours L0 L1 L2 L3 L4 | L5 L6 L9 L12 L38 L58 L61 | L5 L6 L7 L13 L58 L59 | L5 L12 L38 L58 L61 | L5 L13 L58 L59 | L12 L13 L38 L59 L60 L61 | L7 L8 L9 L12 L13 L38 L59 L60 L61 | L14 L15 L16 L17 | L20 L21 L22 L23 | L26 L29 L32 L33 L34 L35 L36 L37 | L26 L27 L28 L29 L33 L35 L36 L37 L41 L42 L43 L44 L47 L48 L49 L51 L52 L55 L56 L57 | L26 L27 L40 L41 L42 L43 L44 L45 | L28 L29 L46 L47 L48 L49 L50 L51 | L27 L28 L52 L53 L54 L55 L56 L57 picked at (23.287847, 31.166667) picked at (-3.5, 20.5) picked at (3.5, 20.5) picked at (-0.166667, 21) picked at (0.166667, 23) picked at (0, 29) picked at (-3.5, 29.5) picked at (-10.833333, 25) picked at (10.833333, 25) picked at (20.121181, 48) picked at (1.666667, 43.166667) picked at (-20.121181, 48) picked at (20.121181, 2) picked at (-21.787847, 3.666667) bodies 6 in component "Spectrometer"
extrude "Extrude18" add sketch "Modular Slit" along normal blind 1.5 separate body contours L0 L1 L2 L3 L4 | L14 L15 L16 L17 | L20 L21 L22 L23 | L26 L29 L32 L33 L34 L35 L36 L37 | L26 L27 L28 L29 L33 L35 L36 L37 L41 L42 L43 L44 L47 L48 L49 L51 L52 L55 L56 L57 | L26 L27 L40 L41 L42 L43 L44 L45 | L28 L29 L46 L47 L48 L49 L50 L51 | L27 L28 L52 L53 L54 L55 L56 L57 picked at (23.287847, 31.166667) picked at (-10.833333, 25) picked at (10.833333, 25) picked at (20.121181, 48) picked at (1.666667, 43.166667) picked at (-20.121181, 48) picked at (20.121181, 2) picked at (-21.787847, 3.666667) makes body 7 in component "Spectrometer"
extrude "Extrude19" add sketch "Modular Slit" along normal blind 4.5 contours L26 L29 L32 L33 L34 L35 L36 L37 | L26 L27 L40 L41 L42 L43 L44 L45 | L28 L29 L46 L47 L48 L49 L50 L51 | L27 L28 L52 L53 L54 L55 L56 L57 picked at (20.121181, 48) picked at (-20.121181, 48) picked at (20.121181, 2) picked at (-21.787847, 3.666667) bodies 7 in component "Spectrometer"
chamfer "Chamfer8" distance 0.5 angle 45 8 edges at (4.5, -22.287847, 4) (4.5, -19.787847, 1.5) (4.5, 19.787847, 1.5) (4.5, 22.287847, 4) (4.5, 22.287847, 46) (4.5, 19.787847, 48.5) (4.5, -19.787847, 48.5) (4.5, -22.287847, 46) on bodies 7 in component "Spectrometer"
chamfer "Chamfer9" distance 0.5 angle 45 6 edges at (1.5, -22.287847, 25.5) (1.5, -15.518924, 1.5) (1.5, -8.75, 4.5) (1.5, 8.75, 4.5) (1.5, 15.518924, 1.5) (1.5, 22.287847, 25.5) on bodies 6 in component "Spectrometer"
extrude "Extrude20" add sketch "Modular Slit" along normal blind 1.5 separate body contours L0 L1 L2 L3 L4 | L5 L6 L9 L12 L38 L58 L61 | L5 L6 L7 L13 L58 L59 | L7 L8 L9 L12 L13 L38 L59 L60 L61 | L14 L15 L16 L17 | L20 L21 L22 L23 | L26 L29 L32 L33 L34 L35 L36 L37 | L26 L27 L28 L29 L33 L35 L36 L37 L41 L42 L43 L44 L47 L48 L49 L51 L52 L55 L56 L57 | L26 L27 L40 L41 L42 L43 L44 L45 | L28 L29 L46 L47 L48 L49 L50 L51 | L27 L28 L52 L53 L54 L55 L56 L57 picked at (23.287847, 31.166667) picked at (-3.5, 20.5) picked at (3.5, 20.5) picked at (-3.5, 29.5) picked at (-10.833333, 25) picked at (10.833333, 25) picked at (20.121181, 48) picked at (1.666667, 43.166667) picked at (-20.121181, 48) picked at (20.121181, 2) picked at (-21.787847, 3.666667) makes body 8 in component "Spectrometer"
extrude "Extrude21" add sketch "Modular Slit" along normal blind 4.5 contours L26 L29 L32 L33 L34 L35 L36 L37 | L26 L27 L40 L41 L42 L43 L44 L45 | L28 L29 L46 L47 L48 L49 L50 L51 | L27 L28 L52 L53 L54 L55 L56 L57 picked at (20.121181, 48) picked at (-20.121181, 48) picked at (20.121181, 2) picked at (-21.787847, 3.666667) bodies 8 in component "Spectrometer"
chamfer "Chamfer10" distance 0.5 angle 45 8 edges at (4.5, -22.287847, 4) (4.5, -19.787847, 1.5) (4.5, 19.787847, 1.5) (4.5, 22.287847, 4) (4.5, 22.287847, 46) (4.5, 19.787847, 48.5) (4.5, -19.787847, 48.5) (4.5, -22.287847, 46) on bodies 8 in component "Spectrometer"
move_face "OffsetFaces1" offset 2 1 faces at (66.883546, 28.871145, 33.333333) on bodies 5 in component "Spectrometer"
move_face "OffsetFaces2" offset 2 1 faces at (64.507313, 27.328001, 50.5) on bodies 4 in component "Spectrometer"
hole "Hole1" at (60.482688, 27.099106, 25) direction (0.544639, -0.838671, 0) diameter 3.416 depth 12 tip angle 118 bodies 5 in component "Spectrometer"
thread "Thread1" "ANSI Unified Screw Threads 0.164(#8) 8-32 UNC 2B" major diameter 4.1656 minor diameter 3.4163 pitch 0.79375 angle 60 modelled right hand crest width 0.234097 on face at (60.835163, 23.660564, 24.344371) crest through (60.590765, 26.932682, 26.70815) on bodies 5 in component "Spectrometer"
extrude "Extrude22" add 1 faces at (6.5, -2.5, 1.5) along direction (0, 0, 1) blind 1 on bodies 1 bodies 1 in component "Spectrometer"
move_body "Move3" [suppressed] in component "Spectrometer"
component "Spectrometer" placed x (1, 0, 0) y (0, 1, 0) z (0, 0, 1) at (0, 0, 0)
hidden bodies 3 6 7 8
equation "d1 = SlitToGrate"
equation "d3 = GrateWidth / 2"
equation "d4 = GrateWidth / 2"
equation "SlitToGrate = 72 mm"
equation "GrateWidth = 51 mm"
equation "GrateAngle = 147 deg"
equation "d9 = 270 deg - GrateAngle"
equation "d10 = ( GrateThickness + GrateTolerance ) / 2"
equation "d11 = ( GrateThickness + GrateTolerance ) / 2"
equation "d12 = GrateWidth"
equation "d13 = GrateThickness + GrateTolerance"
equation "d14 = GrateWidth"
equation "GrateThickness = 1 mm"
equation "GrateTolerance = 0.2 mm"
equation "BoxOuterWidth = ( ( ( GrateWidth + 2 * GrateHolderThickness ) / 2 ) * sin(GrateAngle - 90 deg) + ( ( ( GrateThickness + GrateTolerance ) / 2 + GrateHolderThickness ) * sin(180 deg - GrateAngle) ) ) * 2"
equation "d18 = BoxOuterWidth / 2"
equation "d19 = BoxOuterWidth / 2"
equation "WallThickness = 1.5 mm"
equation "GrateHolderThickness = 1.5 mm"
equation "d22 = ( GrateThickness + GrateTolerance ) / 2 + GrateHolderThickness"
equation "d23 = GrateWidth / 2 + GrateHolderThickness"
equation "d24 = GrateThickness + GrateTolerance + GrateHolderThickness * 2"
equation "d26 = GrateWidth + GrateHolderThickness * 2"
equation "d27 = GrateThickness + GrateTolerance + GrateHolderThickness * 2"
equation "d28 = GrateWidth / 2 + GrateHolderThickness"
equation "d29 = WallThickness"
equation "d30 = BoxOuterWidth / 2 - WallThickness"
equation "d32 = BoxOuterWidth / 2 - WallThickness"
equation "CuvetteSide = 15 mm"
equation "d34 = CuvetteSide"
equation "d35 = CuvetteSide / 2"
equation "d36 = CuvetteSide"
equation "d37 = CuvetteSide / 2"
equation "d38 = CuvetteSide"
equation "CuvetteWallThickness = 1.25 mm"
equation "d40 = CuvetteWallThickness"
equation "d41 = CuvetteSide / 2 + CuvetteWallThickness"
equation "d42 = CuvetteSide + CuvetteWallThickness"
equation "d43 = CuvetteSide / 2 + CuvetteWallThickness"
equation "d44 = CuvetteSide + CuvetteWallThickness"
equation "SlitWidth = 1 mm"
equation "d46 = SlitWidth / 2"
equation "d47 = WallThickness"
equation "d48 = SlitWidth / 2"
equation "d49 = WallThickness"
equation "d50 = SlitWidth"
equation "GrateHolderBuffer = 5 mm"
equation "d52 = GrateHolderBuffer"
equation "d53 = ( GrateThickness + GrateTolerance ) / 2 + GrateHolderThickness"
equation "d54 = ( GrateThickness + GrateTolerance ) / 2 + GrateHolderThickness"
equation "d55 = GrateHolderBuffer"
equation "d56 = ( GrateThickness + GrateTolerance ) / 2 + GrateHolderThickness"
equation "d57 = ( GrateThickness + GrateTolerance ) / 2 + GrateHolderThickness"
equation "SlitHeight = 12 mm"
equation "BoxOuterHeight = 50 mm"
equation "CuvetteHolderHeight = 5 mm"
equation "FoldingInterface = 0.5 mm"
equation "d62 = BoxOuterHeight"
equation "d63 = BoxOuterWidth / 2"
equation "d64 = BoxOuterWidth / 2"
equation "d65 = BoxOuterHeight"
equation "d66 = BoxOuterHeight"
equation "d67 = BoxOuterWidth"
equation "d68 = WallThickness"
equation "d70 = GrateWidth / 2 + GrateHolderThickness"
equation "d71 = BoxOuterHeight / 2"
equation "CamInnerSeparation = 39.6 mm"
equation "d74 = CamInnerSeparation / 2"
equation "CamPeg = 2.4 mm"
equation "CamPegTol = 0.1 mm"
equation "d80 = CamPeg + CamPegTol"
equation "CamInOut = 4.24 mm"
equation "d82 = CamInOut"
equation "d83 = CamPeg + CamPegTol"
equation "CamWidth = 39 mm"
equation "d87 = CamWidth"
equation "d88 = CamWidth"
equation "d89 = GrateWidth + 2 * GrateHolderThickness"
equation "d90 = BoxOuterHeight"
equation "CamPegBase = 3.5 mm"
equation "d92 = CamPegBase"
equation "d93 = CamPegBase"
equation "d96 = 3.5 mm + ( 7.5 / 2 ) * 1 mm"
equation "d102 = WallThickness"
equation "d104 = BoxOuterHeight"
equation "d106 = WallThickness + CuvetteHolderHeight + CuvetteBaseHeight"
equation "d108 = ( BoxOuterHeight - SlitHeight ) / 2"
equation "d109 = SlitHeight"
equation "d111 = WallThickness"
equation "d113 = WallThickness + PegBaseHeight"
equation "PegBaseHeight = 1.5 mm"
equation "PegHeight = 2.5 mm"
equation "d117 = WallThickness + PegBaseHeight + PegHeight"
equation "d120 = BoxOuterHeight / 2"
equation "d121 = GrateWidth + 2 * WallThickness"
equation "d122 = BoxOuterHeight"
equation "d123 = GrateWidth"
equation "d124 = BoxOuterHeight - 2 * WallThickness"
equation "d125 = -WallThickness + PegBaseHeight + CamDistance - CamBuffer"
equation "CamDistance = 28 mm"
equation "d128 = CamDistance + GrateHolderThickness * 2 + GrateThickness + GrateTolerance - WallThickness"
equation "d129 = BoxOuterHeight"
equation "d130 = WallThickness"
equation "d133 = -WallThickness"
equation "d136 = -CuvetteHolderHeight * 2"
equation "d141 = CamBuffer"
equation "d144 = CamBuffer"
equation "d148 = CamBuffer"
equation "d152 = CamBuffer * 2"
equation "d156 = CamInnerSeparation / 2 - CamPeg"